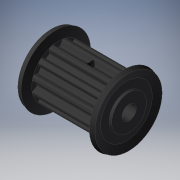
# Autodesk Inventor part: TTPS12T5200-A-P5_b
Saved by Autodesk Inventor 2019 (Build 230136000, 136)
## iProperties
Created: 2023-11-09
Part Number: TTPS12T5200-A-P5_b
Material: Generic
Catalog Web Link: www.cadenas.de
Description: TTPA__T5050, TTPA__T5100, TTPA__T5150, TTPA__T5200, TTPA__T5250, TTPB__T5050, TTPB__T5100, TTPB__T5150, TTPB__T5200, TTPB__T5250, TTPK__T5050, TTPK__T5100, TTPK__T5150, TTPK__T5200, TTPK__T5250, TTPN__T5050, TTPN__T5100, TTPN__T5150, TTPN__T5200, TTPN__T5250, TTPT__T5050, TTPT__T5100, TTPT__T5150, TTPT__T5200, TTPT__T5250, TTPM__T5050, TTPM__T5100, TTPM__T5150, TTPM__T5200, TTPM__T5250, TTPP__T5050, TTPP__T5100, TTPP__T5150, TTPP__T5200, TTPP__T5250, TTPS__T5050, TTPS__T5100, TTPS__T5150, TTPS__T5200, TTPS__T5250_b-Timing Pulleys T5 Type
Vendor: MISUMI
Document SubType Name: Modeling
Designer: psAdmin
Manufacturer: MISUMI
Mass: 5.68782 g
Surface Area: 38.2091 cm^2
Volume: 5.68782 cm^3
Density: 1 g/cm^3
Appearance: PSOLRGB-175-175-175
Category: PARTsolutions
Company: MISUMI
Title: TTPS12T5200-A-P5
Author: Cadenas PARTsolutions
Comments: Timing Pulleys T5 Type
PSOL_IDENT_0: {$CADENAS_DATA/23d-libs/misumi/metric/51_timing_pulleys/ttpt_t5/ttpa_t5.prj},937 {VTYP=3D},{NB=TTPS1
PSOL_IDENT_1: 2T5200-A-P5_b},{LINA=TTPS12T5200-A-P5},{NN=TTPA__T5050, TTPA__T5100, TTPA__T5150, TTPA__T5200, TTPA_
PSOL_IDENT_2: _T5250, TTPB__T5050, TTPB__T5100, TTPB__T5150, TTPB__T5200, TTPB__T5250, TTPK__T5050, TTPK__T5100, T
PSOL_IDENT_3: TPK__T5150, TTPK__T5200, TTPK__T5250, TTPN__T5050, TTPN__T5100, TTPN__T5150, TTPN__T5200, TTPN__T525
PSOL_IDENT_4: 0, TTPT__T5050, TTPT__T5100, TTPT__T5150, TTPT__T5200, TTPT__T5250, TTPM__T5050, TTPM__T5100, TTPM__
PSOL_IDENT_5: T5150, TTPM__T5200, TTPM__T5250, TTPP__T5050, TTPP__T5100, TTPP__T5150, TTPP__T5200, TTPP__T5250, TT
PSOL_IDENT_6: PS__T5050, TTPS__T5100, TTPS__T5150, TTPS__T5200, TTPS__T5250_b},{DATE=29.05.2023 09:16:51},{GEOMDAT
PSOL_IDENT_7: E=15.12.2022 08:47:30},{VERSION=},{LINEID=10},{WBVAR=MATP,ST,TNW,PS,SBS,DD,Z,J,Q,R,S,T,ALT1,ALT2,M,Q
PSOL_IDENT_8: SC,QFC,QTC,ALT3,K,KSC,KFC,KTC,ALT4,ZM,ZSC,ZFC,ZTC,ALT5,ALT6,ALT7,FC,ALT8,SRG,ALT9,BTC,TL,ALT10,TPC,A
PSOL_IDENT_9: LT11,BC,ALT12,SLH,ALT13,BN},{WBNUMERIC=DD,Z,J,Q,R,S,T,QSC,QFC,QTC,K,KSC,KFC,KTC,ZSC,ZFC,ZTC,FC,SRG,B
PSOL_IDENT_10: TC,TL,BC,SLH,BN}  {NB=TTPS12T5200-A-P5_b},{LINA=TTPS12T5200-A-P5},{KT=DUMMY},{PN=TTPS12T5200-A-P5},{
PSOL_IDENT_11: TYPE=TTPS},{MATP=SUS304},{MATPALG= 'A2017','Aluminum Alloy 2000 series','S45C','1045 Carbon Steel Eq
PSOL_IDENT_12: uivalent','SUS304','304 Stainless Steel' },{ST=-},{STALG= '-','-' },{NT=12},{TNW=T5200},{TNWALG= 'T5
PSOL_IDENT_13: 100' , 'T5150' , 'T5200' , 'T5250' },{BW=20},{PS=A},{PSALG= 'A' },{SBS=P},{SBSALG= 'H','Round Hole','
PSOL_IDENT_14: P','Round Hole + Tap','N','New JIS Keywayed Bore + Tap (Standard)','V','Stepped Hole','Y','Both Ends
PSOL_IDENT_15: Stepped Hole' },{DD=5.00},{DDALG=[5:6/1],6.35,[7:8/1]},{DDHA=[5:6/1],6.35,[7:8/1]},{DDPA=[5:6/1],6.
PSOL_IDENT_16: 35,[7:8/1]},{DDNA=[8:8/1]},{DDCA=},{DDVA=[5:6/1]},{DDY=[5:6/1]},{DDWB=},{DDHB=},{DDPB=},{DDNB=},{DDN
PSOL_IDENT_17: K=[10:10/1]},{DDCB=},{DDVFB=},{Z=0},{ZALG=[0]},{ZMIN=7.000},{ZAMAX=8.000},{ZBMAX=0.000},{DDZ=5.000},
PSOL_IDENT_18: {J=0.0},{JALG=[0]},{JMIN=2.000},{JMAX=25.000},{JPN=},{Q=0},{QALG=[0]},{QRMIN=7.000},{QRMAX=8.000},{W
PSOL_IDENT_19: BQMIN=9.000},{R=0},{RALG=[0]},{WBRMAX=-2.000},{S=0.0},{SALG=[0]},{SMAX=14.000},{T=0.0},{TALG=[0]},{T
PSOL_IDENT_20: MAX=14.000},{SBSPN=-P5},{A=22},{W=27},{L=0},{PD=19.10},{OD=18.25},{D=0},{DALG=0.000},{DE=12.000},{F=
PSOL_IDENT_21: 24},{E=12},{TT=1.6},{BBK=0.000},{TTK=0.000},{ALT1=},{ALT1ALG= '','w/o KC90 (Set Screw Angle)','KC90'
PSOL_IDENT_22: ,'with KC90 (Set Screw Angle)' },{ANG=120.000},{ALT1PN=},{ALT2=},{ALT2ALG= '','Not applicable' },{M=
PSOL_IDENT_23: N/A},{MALG= 'N/A' },{MFTALG= 'N/A' },{MSALG= 'N/A' },{M3D=0.000},{KDML=0.000},{ML=0.000},{MUL=0.000}
PSOL_IDENT_24: ,{PITCH=0.000},{QSC=0.0},{QSCALG=0},{QFC=0.0},{QFCALG=0},{QTC=0.0},{QTCALG=0},{QPCDMIN=0.000},{QPCDM
PSOL_IDENT_25: INALG=0.000},{QPCDMAX=8.000},{ALT2PN=},{TAP=0.000},{ALT3=},{ALT3ALG= '','Not applicable' },{K=0.0},{
PSOL_IDENT_26: KALG=0},{KMIN=4.000},{KFTMAX=0.000},{KSMAX=0.000},{KSC=0.0},{KSCALG=0},{KFC=0.0},{KFCALG=0},{KTC=0.0
PSOL_IDENT_27: },{KTCALG=0},{KSCMIN=9.000},{KPCDMIN=9.000},{KPCDMAX=8.000},{ALT3PN=},{ALT4=},{ALT4ALG= '','Not appl
PSOL_IDENT_28: icable' },{ALT4MIN=15.500},{ALT4MAX=1.500},{ZM=N/A},{ZMALG= 'N/A' },{ZMFTALG= 'N/A' },{ZMSALG= 'N/A'
PSOL_IDENT_29: },{ZMDD1=0.0},{ZMDD2=0.0},{ZMHH=0.0},{ZSC=0.0},{ZSCALG=[0]},{ZFC=0.0},{ZFCALG=[0]},{ZTC=0.0},{ZTCAL
PSOL_IDENT_30: G=[0]},{ZPCDMIN=0.000},{ZPCDMINALG=0.000},{ZPCDMAX=8.000},{ALT4PN=},{ALT5=},{ALT5ALG= '','w/o Flange
PSOL_IDENT_31: not Attached','NFC','with NFC (Flange not Attached)' },{ALT5PN=},{ALT6=},{ALT6ALG= '','w/o Flange A
PSOL_IDENT_32: ttached on One Side Only','RFC','with RFC (Flange Attached on The Boss Side Only)','LFC','with LFC (
PSOL_IDENT_33: Flange Attached on The Opposite Side Only)' },{ALT6PN=},{ALT7=},{ALT7ALG= '','w/o FC (Flange Cut)','
PSOL_IDENT_34: FC','with FC (Flange Cut)' },{FC=0.0},{FCALG=0},{FCMIN=19.5},{FCMAX=22.0},{ALT7PN=},{ALT8=},{ALT8ALG=
PSOL_IDENT_35: '','Not applicable' },{ALT8ALGALG=8.000},{ALT8DD2=0.000},{ALT8MM=0.000},{ALT8NN=0.000},{QC=0.000},{
PSOL_IDENT_36: KC=0.000},{ZC=0.000},{SRG=0.0},{SRGALG=[0]},{SRGMAX=0.000},{SRGMAX1=0.000},{DD2=0.0},{MM=0.00},{NN=0
PSOL_IDENT_37: .00},{ALT8PN=},{ALT9=},{ALT9ALG= '','Not applicable' },{BTC9=7.000},{TL9=1.000},{BTC=0},{BTCALG=[0]}
PSOL_IDENT_38: ,{TL=0.0},{TLALG=0},{TLMIN=1.000},{TLMAX=-27.500},{BTCL=0},{BTCD=0},{ALT9PN=},{WLBCTL=27.000},{ALT10=
PSOL_IDENT_39: },{ALT10ALG= '','w/o TPC (Tapped Hole Dimension)','TPC','with TPC (Tapped Hole Dimension)' },{TPC=N/
PSOL_IDENT_40: A},{TPCALG= 'N/A' },{TPCM=3.000},{ALT10PN=},{ALT11=},{ALT11ALG= '','Not applicable' },{BC=0.0},{BCAL
PSOL_IDENT_41: G=0},{BCMIN=6.000},{BCMAX=-27.500},{M1WBC=13.500},{ALT11PN=},{KTT=6.625},{ALT12=},{ALT12ALG= '','w/o
PSOL_IDENT_42: SLH (Set Screw Length)','SLH','with SLH (Set Screw Length)' },{SLH=0},{SLHALG=[0]},{ALT12PN=},{AC=M
PSOL_IDENT_43: 3x3},{M1=3.000},{M1L=3.000},{ALT811SRG3D=1.000},{ALT13=},{ALT13ALG= '', 'Not applicable' },{BN=0.0},
PSOL_IDENT_44: {BNALG=0},{BNMIN=-26.5},{BNMAX=-17.0},{ALT13PN=}
NB: TTPS12T5200-A-P5_b
NN: 0
NT: 12
NBSYN: $PN._b
LINA: TTPS12T5200-A-P5
CATALOG: Misumi
PN: TTPS12T5200-A-P5
MATP: 304 Stainless Steel
ST: -
TNW: T5200
BW: 20
PS: A
SBS: Round Hole + Tap
DD: 5
Z: 0
J: 0
Q: 0
R: 0
S: 0
T: 0
A: 22
W: 27
L: 0
PD: 19.1
OD: 18.25
D: 0
F: 24
E: 12
TT: 1.6
ALT1: w/o KC90 (Set Screw Angle)
ALT2: Not applicable
M: N/A
QSC: 0
QFC: 0
QTC: 0
ALT3: Not applicable
K: 0
KSC: 0
KFC: 0
KTC: 0
ALT4: Not applicable
ZM: N/A
ZMDD1: 0
ZMDD2: 0
ZMHH: 0
ZSC: 0
ZFC: 0
ZTC: 0
ALT5: w/o Flange not Attached
ALT6: w/o Flange Attached on One Side Only
ALT7: w/o FC (Flange Cut)
FC: 0
ALT8: Not applicable
SRG: 0
DD2: 0
MM: 0
ALT9: Not applicable
BTC: 0
TL: 0
BTCL: 0
BTCD: 0
ALT10: w/o TPC (Tapped Hole Dimension)
TPC: N/A
ALT11: Not applicable
BC: 0
ALT12: w/o SLH (Set Screw Length)
SLH: 0
AC: M3x3
ALT13: Not applicable
BN: 0
SUPPLIER: MISUMI
ARTICLENO: TTPS12T5200-A-P5_b
BOMINFO: TTPS12T5200-A-P5
CREATOR: CADENAS GmbH
Autodesk Inventor part; units mm, degrees
note: some values were not read from the file. Chosen so that the rebuilt part matches the saved one: pattern direction of "Circular Pattern1".
sketch "_____2" plane through (0, 0, 0) normal (0, 0, 1) x (1, 0, 0)
  line L0 (27, 0) -> (0, 0)
  line L1 (0, 0) -> (0, 6)
  line L2 (0, 6) -> (0.9, 6)
  line L3 (0.9, 6) -> (0.9, 8.9144)
  line L4 (0.9, 8.9144) -> (0.1842, 11.5859)
  line L5 (0.1842, 11.5859) -> (1.7296, 12)
  line L6 (1.7296, 12) -> (2.5, 9.125)
  line L7 (2.5, 9.125) -> (24.5, 9.125)
  line L8 (24.5, 9.125) -> (25.2704, 12)
  line L9 (25.2704, 12) -> (26.8158, 11.5859)
  line L10 (26.8158, 11.5859) -> (26.1, 8.9144)
  line L11 (26.1, 8.9144) -> (26.1, 6)
  line L12 (26.1, 6) -> (27, 6)
  line L13 (27, 6) -> (27, 0)
  line L14 (27, 0) -> (0, 0)
  constraints: 30 end point
revolve "Revolution1" add sketch "_____2" angle 360 about axis through (27, 0, 0) along (1, 0, 0)
sketch "Sketch2" plane through (27, 0, 0) normal (1, 0, 0) x (0, 0, -1)
  point P0 (0, 0)
hole "Hole1" at (27, 0, 0) direction (-1, 0, 0) diameter 5 depth 27
sketch "_____6" plane through (2.5, 0, 0) normal (1, 0, 0) x (0, 0, -1)
  line L0 (-2.1179, 9.3122) -> (-2.0236, 8.8978)
  arc A0 (-1.3468, 8.5663) -> (-2.0236, 8.8978) centre (-1.8906, 8.3127) ccw
  line L1 (-1.3468, 8.5663) -> (-0.8679, 7.5394)
  arc A1 (-0.8679, 7.5394) -> (-0.4792, 7.3093) centre (-0.5054, 7.7084) ccw
  arc A2 (0.4792, 7.3093) -> (-0.4792, 7.3093) centre (0, 0) ccw
  arc A3 (0.4792, 7.3093) -> (0.8679, 7.5394) centre (0.5054, 7.7084) ccw
  line L2 (0.8679, 7.5394) -> (1.3468, 8.5663)
  arc A4 (2.0236, 8.8978) -> (1.3468, 8.5663) centre (1.8906, 8.3127) ccw
  line L3 (2.0236, 8.8978) -> (2.1179, 9.3122)
  arc A5 (2.1179, 9.3122) -> (-2.1179, 9.3122) centre (0, 0) ccw
  constraints: 12 point on circle, 8 end point, 6 centre point
extrude "Extrusion1" cut sketch "_____6" along normal blind 22
pattern_circular "Circular Pattern1" count 12 over 360 about axis through (2.5, 0, 0) along (1, 0, 0) of "Extrusion1"
sketch "_____15" plane through (13.5, 0, 0) normal (1, 0, 0) x (0, 0, -1)
  line L0 (0, 0) -> (0, 9.125)
  line L1 (0, 9.125) -> (1.2295, 9.125)
  line L2 (1.2295, 9.125) -> (1.2295, 0)
  line L3 (1.2295, 0) -> (0, 0)
  line L4 (0, 0) -> (0, 9.125)
  constraints: 10 end point
revolve "Revolution2" cut sketch "_____15" angle 360 about axis through (13.5, 0, 0) along (0, -1, 0)
thread "Thread1" size "M3x0.5" class "6H" standard "ISO Metric profile" length 6.625
sketch "_____16" plane through (13.5, 0, 0) normal (1, 0, 0) x (0, 0, -1)
  line L0 (0, 0) -> (7.9025, -4.5625)
  line L1 (7.9025, -4.5625) -> (7.2877, -5.6273)
  line L2 (7.2877, -5.6273) -> (-0.6148, -1.0648)
  line L3 (-0.6148, -1.0648) -> (0, 0)
  line L4 (0, 0) -> (7.9025, -4.5625)
  constraints: 10 end point
revolve "Revolution3" cut sketch "_____16" angle 360 about axis through (13.5, 0, 0) along (0, 0.5, 0.8660254)
thread "Thread2" size "M3x0.5" class "6H" standard "ISO Metric profile" length 6.625
ref_plane "to_screw1_XY" through (13.5, 2.5, 0) normal (0, 1, 0) x (1, 0, 0)
ref_plane "to_screw1_YZ" through (13.5, 2.5, 0) normal (1, 0, 0) x (0, 0, -1)
ref_plane "to_screw1_ZX" through (13.5, 2.5, 0) normal (0, 0, -1) x (0, 1, 0)
ref_plane "to_screw2_XY" through (13.5, -1.25, -2.1651) normal (0, -0.5, -0.8660254) x (1, 0, 0)
ref_plane "to_screw2_YZ" through (13.5, -1.25, -2.1651) normal (1, 0, 0) x (0, -0.8660254, 0.5)
ref_plane "to_screw2_ZX" through (13.5, -1.25, -2.1651) normal (0, -0.8660254, 0.5) x (0, -0.5, -0.8660254)
body "Solid1"
